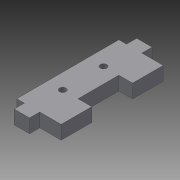
# Autodesk Inventor part: Frame_Lower_Vertical_Plate_A
Saved by Autodesk Inventor 2014 (Build 180170000, 170)
## iProperties
Created: 2014-08-27
Part Number: Frame_Lower_Vertical_Plate_A
Material: Generic
Document SubType Name: Modeling
Designer: ThatOtherGuy
Density: 1 g/cm^3
Appearance: Default
Author: ThatOtherGuy
Autodesk Inventor part; units mm, degrees
ref_plane "YZ Plane" through (0, 0, 0) normal (1, 0, 0) x (0, 1, 0)
ref_plane "XZ Plane" through (0, 0, 0) normal (0, 1, 0) x (-1, 0, 0)
ref_plane "XY Plane" through (0, 0, 0) normal (0, 0, 1) x (1, 0, 0)
sketch "Sketch1" plane through (0, 0, 0) normal (0, 0, 1) x (1, 0, 0)
  line L0 (0, 0) -> (3.75, 0)
  line L1 (3.75, 0) -> (3.75, -5)
  line L2 (3.75, -5) -> (11.25, -5)
  line L3 (11.25, -5) -> (11.25, 0)
  line L4 (11.25, 0) -> (21.731, 0)
  line L5 (21.731, 0) -> (21.731, 50)
  line L6 (21.731, 50) -> (11.25, 50)
  line L7 (11.25, 50) -> (11.25, 55)
  line L8 (11.25, 55) -> (3.75, 55)
  line L9 (3.75, 55) -> (3.75, 50)
  line L10 (3.75, 50) -> (0, 50)
  line L11 (0, 50) -> (0, 0)
  line L12 (21.731, 35) -> (15, 35)
  line L13 (15, 35) -> (15, 15)
  line L14 (15, 15) -> (21.731, 15)
  line L15 (21.731, 15) -> (21.731, 35)
  circle A0 centre (7.5, 35) radius 1.6
  circle A1 centre (7.5, 15) radius 1.6
  line L16 (7.5, 15) -> (7.5, 35)
  point P0 (21.731, 25)
  point P1 (21.731, 25)
  point P2 (7.5, -5)
  point P3 (7.5, 25)
  point P4 (0, 25)
  dimension "d0" = 50
  dimension "d1" = 3.75
  dimension "d2" = 5
  dimension "d3" = 7.5
  dimension "d4" = 10.481
  dimension "d5" = 6.731
  dimension "d6" = 20
  dimension "d7" = 3.75
  dimension "d10" = 3.2
  dimension "d11" = 20
  constraints: 34 end point, 10 parallel, 5 equal length, 5 midpoint, 2 centre point, 2 collinear, 2 horizontal, 2 perpendicular, 2 vertical alignment, 1 coincident, 1 equal radius, 1 horizontal alignment
  measures "d0" distance of L10.end L0.start
  measures "d1" distance of L0.start L0.end
  measures "d2" distance of L0.end L1.end
  measures "d3" distance of L7.end L8.end
  measures "d4" distance of L5.end L6.end
  measures "d5" distance of L12.start L12.end
  measures "d6" distance of L12.end L13.end
  measures "d7" distance between parallel lines of L3 L13
  measures "d10" diameter of A0
  measures "d11" distance of L16.start L16.end
extrude "Extrusion1" add sketch "Sketch1" along normal blind 6.731 contours L11 L10 L9 L8 L7 L6 L5 L12 L13 L14 L4 L3 L2 L1 L0
equation "\"d4\" = d7 + THICKB"
equation "\"d5\" = THICKB"
equation "\"d7\" = d1"
equation "\"d8\" = THICKB"
equation "\"THICKA\" = 3.175"
equation "\"THICKB\" = 6.731"
equation "\"THICKC\" = 12.7"
equation "\"BALLDIA\" = 12"
equation "\"MAGDIA\" = 9.5"
equation "\"THICKPLY\" = 5"
body "Solid1"
